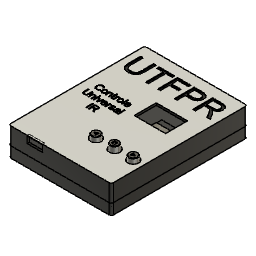
NOVACASEEMBARCADOS v11 (Autodesk Fusion 360 design; units mm, degrees)
Autodesk Fusion 360 part; units mm, degrees
sketch "Esboço1" plane through (0, 0, 0) normal (0, 0, 1) x (1, 0, 0)
  line L0 (-44.75, 0) -> (-44.75, 60)
  line L1 (-44.75, 0) -> (-44.75, -60)
  line L2 (-44.75, -60) -> (44.75, -60)
  line L3 (44.75, -60) -> (44.75, 60)
  line L4 (44.75, 60) -> (-44.75, 60)
  dimension "d2" = 44.75
  dimension "d3" = 60
  dimension "d4" = 60
  dimension "d5" = 89.5
  constraint perpendicular L1 L2
  constraint perpendicular L2 L3
  constraint perpendicular L0 L4
  measures "d2" distance of origin L0.start
  measures "d3" distance of L0.start L0.end
  measures "d4" distance of L0.start L1.end
  measures "d5" distance of L1.end L2.end
extrude "Extrusão1" add sketch "Esboço1" along normal blind 1.5 makes body 1
sketch "Esboço2" plane through (0, 0, 1.5) normal (0, 0, 1) x (-1, 0, 0)
  line L0 (44.75, -60) -> (44.75, 60)
  line L1 (44.75, 60) -> (-44.75, 60)
  line L2 (-44.75, 60) -> (-44.75, -60)
  line L3 (-44.75, -60) -> (44.75, -60)
  line L4 (-40.75, 36) -> (-34.75, 36)
  line L5 (-40.75, 36) -> (-40.75, 30)
  line L6 (-34.75, 36) -> (-34.75, 30)
  line L7 (-34.75, 30) -> (-40.75, 30)
  line L8 (-23.75, 36) -> (-17.75, 36)
  line L9 (-23.75, 36) -> (-23.75, 30)
  line L10 (-17.75, 36) -> (-17.75, 30)
  line L11 (-17.75, 30) -> (-23.75, 30)
  line L12 (-0.75, 30) -> (-6.75, 30)
  line L13 (-6.75, 36) -> (-6.75, 30)
  line L14 (-6.75, 36) -> (-0.75, 36)
  line L15 (-0.75, 36) -> (-0.75, 30)
  line L16 (-31.75, 0) -> (-3.75, 0)
  line L17 (-3.75, 0) -> (-3.75, -27)
  line L18 (-31.75, 0) -> (-31.75, -27)
  line L19 (-31.75, -27) -> (-3.75, -27)
  line L20 (36.75, 57) -> (8.75, 57)
  line L21 (8.75, 57) -> (8.75, 6)
  line L22 (36.75, 57) -> (36.75, 6)
  line L23 (36.75, 6) -> (8.75, 6)
  dimension "d10" = 6
  dimension "d11" = 6
  dimension "d12" = 11
  dimension "d13" = 6
  dimension "d15" = 6
  dimension "d18" = 28
  dimension "d19" = 27
  dimension "d22" = 28
  dimension "d23" = 51
  constraint perpendicular L4 L5
  constraint perpendicular L4 L6
  constraint perpendicular L5 L7
  constraint perpendicular L8 L10
  constraint perpendicular L9 L11
  constraint perpendicular L14 L15
  constraint perpendicular L12 L13
  constraint perpendicular L17 L19
  constraint perpendicular L20 L21
  constraint perpendicular L20 L22
  constraint perpendicular L21 L23
  measures "d10" distance of L4.start L4.end
  measures "d11" distance of L4.start L5.end
  measures "d12" distance of L4.end L8.start
  measures "d13" distance of L8.start L8.end
  measures "d15" distance of L13.start L14.end
  measures "d18" distance of L16.start L16.end
  measures "d19" distance of L16.end L17.end
  measures "d22" distance of L20.start L20.end
  measures "d23" distance of L20.end L21.end
extrude "Extrusão2" add sketch "Esboço2" along normal blind 16.5 contours L20 L21 L22 L23 bodies 1
extrude "Extrusão3" add sketch "Esboço2" along normal blind 3.5 contours L16 L17 L18 L19 bodies 1
extrude "Extrusão4" add sketch "Esboço2" along normal blind 3.5 contours L4 L5 L6 L7 | L8 L9 L10 L11 | L12 L13 L14 L15 bodies 1
sketch "Esboço3" plane through (0, 0, 5) normal (0, 0, 1) x (-1, 0, 0)
  line L0 (-31.75, 0) -> (-31.75, -27)
  line L1 (-31.75, -27) -> (-3.75, -27)
  line L2 (-3.75, -27) -> (-3.75, 0)
  line L3 (-3.75, 0) -> (-31.75, 0)
  line L4 (-29.75, -4.5) -> (-5.25, -4.5)
  line L5 (-5.25, -4.5) -> (-5.25, -20.5)
  line L6 (-5.25, -20.5) -> (-29.75, -20.5)
  line L7 (-29.75, -20.5) -> (-29.75, -4.5)
  dimension "d32" = 24.5
  dimension "d33" = 16
  constraint perpendicular L4 L5
  constraint perpendicular L4 L7
  measures "d32" distance of L4.start L4.end
  measures "d33" distance of L4.end L5.end
extrude "Extrusão5" add sketch "Esboço3" along normal blind 2 contours L4 L5 L6 L7 bodies 1
sketch "Esboço4" plane through (0, 0, 1.5) normal (0, 0, 1) x (-1, 0, 0)
sketch "Esboço5" plane through (0, 0, 5) normal (0, 0, 1) x (-1, 0, 0)
  line L0 (-40.75, 36) -> (-40.75, 30)
  line L1 (-40.75, 30) -> (-34.75, 30)
  line L2 (-34.75, 30) -> (-34.75, 36)
  line L3 (-34.75, 36) -> (-40.75, 36)
  circle A0 centre (-3.75, 33) radius 1.5
  circle A1 centre (-20.75, 33) radius 1.5
  circle A2 centre (-37.75, 33) radius 1.5
  dimension "d40" = 3
  dimension "d41" = 3
  dimension "d42" = 3
  measures "d40" diameter of A0
  measures "d41" diameter of A1
  measures "d42" diameter of A2
extrude "Extrusão6" add sketch "Esboço5" along normal blind 2 contours A0 | A2 bodies 1
extrude "Extrusão7" add sketch "Esboço5" along normal blind 3 contours A1 bodies 1
chamfer "Chanfro1" distance 0.25 distance2 3 1 edges at (22.1485, -32.4576, 8) measured on face at (20.7773, -33.3643, 8) on bodies 1
sketch "Esboço7" plane through (0, -57, 0) normal (0, -1, 0) x (1, 0, 0)
  line L0 (-36.75, 1.5) -> (-8.75, 1.5)
  line L1 (-8.75, 1.5) -> (-8.75, 18)
  line L2 (-8.75, 18) -> (-36.75, 18)
  line L3 (-36.75, 18) -> (-36.75, 1.5)
  line L4 (-26.75, 18) -> (-19.75, 18)
  line L5 (-27.75, 17) -> (-26.75, 18)
  line L6 (-27.75, 17) -> (-26.25, 16)
  line L7 (-26.25, 16) -> (-21.25, 16)
  line L8 (-19.75, 18) -> (-18.75, 17)
  line L9 (-18.75, 17) -> (-20, 16)
  line L10 (-20, 16) -> (-21.25, 16)
  line L11 (-27.75, 17) -> (-26.25, 16)
  dimension "d49" = 10
  dimension "d50" = 7
  dimension "d55" = 5
  constraint parallel L2 L4
  constraint horizontal L7
  measures "d49" distance of L2.end L4.start
  measures "d50" distance of L4.start L4.end
  measures "d55" distance of L6.end L7.end
extrude "Extrusão8" cut sketch "Esboço7" against normal blind 5 contours L2 L4 L5 L6 L7 L8 L9 L10 L11 bodies 1
sketch "Esboço8" plane through (0, 0, 1.5) normal (0, 0, 1) x (-1, 0, 0)
sketch "Esboço9" plane through (0, 0, 0) normal (0, 0, 1) x (1, 0, 0)
  line L0 (164.75, -60) -> (75.25, -60)
  line L1 (75.25, -60) -> (75.25, 60)
  line L2 (164.75, 60) -> (164.75, -60)
  line L3 (75.25, 60) -> (164.75, 60)
  line L4 (73.25, -62) -> (73.25, 62)
  line L5 (73.25, 62) -> (166.75, 62)
  line L6 (166.75, 62) -> (166.75, -62)
  line L7 (166.75, -62) -> (73.25, -62)
  dimension "d61" = -2
  constraint horizontal L3
  constraint vertical L2
  constraint horizontal L0
  constraint vertical L1
extrude "Extrusão9" add sketch "Esboço9" along normal blind 2 separate body contours L0 L1 L2 L3 makes body 2
extrude "Extrusão11" add sketch "Esboço9" along normal blind 9.75 bodies 2
sketch "Esboço10" plane through (0, 0, 9.75) normal (0, 0, 1) x (-1, 0, 0)
  line L0 (-75.25, 60) -> (-75.25, -60)
  line L1 (-75.25, -60) -> (-164.75, -60)
  line L2 (-164.75, -60) -> (-164.75, 60)
  line L3 (-164.75, 60) -> (-75.25, 60)
  line L4 (-166.75, 62) -> (-166.75, -62)
  line L5 (-166.75, -62) -> (-73.25, -62)
  line L6 (-73.25, -62) -> (-73.25, 62)
  line L7 (-73.25, 62) -> (-166.75, 62)
  line L8 (-74.25, 61) -> (-74.25, -61)
  line L9 (-74.25, -61) -> (-165.75, -61)
  line L10 (-165.75, -61) -> (-165.75, 61)
  line L11 (-165.75, 61) -> (-74.25, 61)
extrude "Extrusão12" cut sketch "Esboço10" against normal blind 3 contours L8 L9 L10 L11 bodies 2
sketch "Esboço11" plane through (0, 0, 0) normal (0, 0, 1) x (1, 0, 0)
  line L0 (203.25, 62) -> (296.75, 62)
  line L1 (296.75, 62) -> (296.75, -62)
  line L2 (296.75, -62) -> (203.25, -62)
  line L3 (203.25, -62) -> (203.25, 62)
  line L4 (294.75, -60) -> (205.25, -60)
  line L5 (205.25, -60) -> (205.25, 60)
  line L6 (205.25, 60) -> (294.75, 60)
  line L7 (294.75, 60) -> (294.75, -60)
  dimension "d71" = 2
  constraint horizontal L0
  constraint vertical L1
  constraint horizontal L2
  constraint vertical L3
extrude "Extrusão13" add sketch "Esboço11" along normal blind 2 separate body contours L4 L5 L6 L7 makes body 3
extrude "Extrusão14" add sketch "Esboço11" along normal blind 12.75 bodies 3
sketch "Esboço12" plane through (0, 0, 12.75) normal (0, 0, 1) x (-1, 0, 0)
  line L0 (-205.25, -60) -> (-294.75, -60)
  line L1 (-294.75, -60) -> (-294.75, 60)
  line L2 (-294.75, 60) -> (-205.25, 60)
  line L3 (-205.25, 60) -> (-205.25, -60)
  line L4 (-203.25, 62) -> (-296.75, 62)
  line L5 (-296.75, 62) -> (-296.75, -62)
  line L6 (-296.75, -62) -> (-203.25, -62)
  line L7 (-203.25, -62) -> (-203.25, 62)
  line L8 (-203.25, -62) -> (-296.75, -62)
  line L9 (-296.75, -62) -> (-296.75, 62)
  line L10 (-296.75, 62) -> (-203.25, 62)
  line L11 (-203.25, 62) -> (-203.25, -62)
  line L12 (-295.75, -61) -> (-295.75, 61)
  line L13 (-295.75, 61) -> (-204.25, 61)
  line L14 (-204.25, 61) -> (-204.25, -61)
  line L15 (-204.25, -61) -> (-295.75, -61)
  dimension "d76" = 1
  constraint horizontal L8
  constraint vertical L9
  constraint horizontal L10
  constraint vertical L11
  constraint coincident L4.end L5.start
  constraint coincident L6.end L7.start
extrude "Extrusão15" cut sketch "Esboço12" against normal blind 3 contours L4 L5 L6 L7 L8 L9 L10 L11 bodies 3
move_body "Alinhar1" bodies 1 to x (1, 0, 0) y (0, 1, 0) z (0, 0, 1) at (120, 0, 0)
move_body "Mover1" bodies 3 to x (-1, 0, 0) y (0, 1, 0) z (0, 0, -1) at (591.5, 0, 25.5)
move_body "Alinhar2" bodies 3 to x (1, 0, 0) y (0, 1, 0) z (0, 0, 1) at (-221.5, 0, -6)
sketch "Esboço13" plane through (0, 0, 19.5) normal (0, 0, 1) x (-1, 0, 0)
  line L0 (-73.25, 62) -> (-166.75, 62)
  line L1 (-166.75, 62) -> (-166.75, -62)
  line L2 (-166.75, -62) -> (-73.25, -62)
  line L3 (-73.25, -62) -> (-73.25, 62)
  line L4 (-151.75, -2.5) -> (-123.25, -2.5)
  line L5 (-123.25, -2.5) -> (-123.25, -22.5)
  line L6 (-123.25, -22.5) -> (-151.75, -22.5)
  line L7 (-151.75, -22.5) -> (-151.75, -2.5)
  circle A0 centre (-123.75, 33) radius 5
  circle A1 centre (-140.75, 33) radius 5
  circle A2 centre (-157.75, 33) radius 5
  dimension "d81" = 10
  dimension "d82" = 10
  dimension "d83" = 10
  measures "d81" diameter of A0
  measures "d82" diameter of A1
  measures "d83" diameter of A2
extrude "Extrusão16" add sketch "Esboço13" against normal blind 2 separate body contours L4 L5 L6 L7 | A0 | A1 | A2 makes body 4 at (140.1411, -30.9517, 19.5) makes body 5 at (157.1411, -30.9517, 19.5) makes body 6 at (132.75, 15.8333, 19.5) makes body 7 at (122.4284, -33.696, 19.5)
extrude "Extrusão17" add 4 faces at (140.1411, -30.9517, 19.5) (122.4284, -33.696, 19.5) (157.1411, -30.9517, 19.5) (132.75, 15.8333, 19.5) along direction (0, 0, -1) blind 2 on bodies 4 5 6 7 bodies 3 4 5 6 7
extrude "Extrusão18" cut sketch "Esboço13" against normal blind 3 contours L4 L5 L6 L7 | A0 | A1 | A2 bodies 3
fillet "Arredondamento1" radius 2 2 edges at (166.75, -62, 4.875) (166.75, -62, 14.625) on bodies 2 3
fillet "Arredondamento2" radius 2 2 edges at (73.25, -62, 4.875) (73.25, -62, 14.625) on bodies 2 3
fillet "Arredondamento3" radius 2 2 edges at (166.75, 62, 4.875) (166.75, 62, 14.625) on bodies 2 3
fillet "Arredondamento4" radius 2 2 edges at (73.25, 62, 4.875) (73.25, 62, 14.625) on bodies 2 3
sketch "Esboço14" plane through (0, 0, 19.5) normal (0, 0, 1) x (-1, 0, 0)
  arc A0 (-75.25, -62) -> (-73.25, -60) centre (-75.25, -60) ccw
  line L0 (-73.25, -60) -> (-73.25, 60)
  arc A1 (-73.25, 60) -> (-75.25, 62) centre (-75.25, 60) ccw
  line L1 (-75.25, 62) -> (-164.75, 62)
  arc A2 (-164.75, 62) -> (-166.75, 60) centre (-164.75, 60) ccw
  line L2 (-166.75, 60) -> (-166.75, -60)
  arc A3 (-166.75, -60) -> (-164.75, -62) centre (-164.75, -60) ccw
  line L3 (-164.75, -62) -> (-75.25, -62)
  circle A4 centre (-140.75, 33) radius 5
  line L4 (-123.25, -2.5) -> (-123.25, -22.5)
  line L5 (-123.25, -22.5) -> (-151.75, -22.5)
  line L6 (-151.75, -22.5) -> (-151.75, -2.5)
  line L7 (-151.75, -2.5) -> (-123.25, -2.5)
  circle A5 centre (-123.75, 33) radius 5
  circle A6 centre (-157.75, 33) radius 5
  line L8 (-78.6403, -28.775) -> (-161.6972, -28.775) construction
  line L9 (-161.6972, -28.775) -> (-161.6972, -57.452) construction
  line L10 (-161.6972, -57.452) -> (-78.6403, -57.452) construction
  line L11 (-78.6403, -57.452) -> (-78.6403, -28.775) construction
  line L12 (-79.2776, 23.0559) -> (-116.8762, 23.0559) construction
  line L13 (-116.8762, 23.0559) -> (-116.8762, -21.9776) construction
  line L14 (-116.8762, -21.9776) -> (-79.2776, -21.9776) construction
  line L15 (-79.2776, -21.9776) -> (-79.2776, 23.0559) construction
  dimension "d98" = 18
  dimension "d99" = 6
  text T0 "UTFPR" font "Arial" height 18 align centre middle in box 83.0569 x 28.6769 at (-78.6403, -28.775) x (-1, 0) y (0, -1) spacing 1 kerned
  text T1 "Controle\nUniversal\nIR" font "Arial" height 6 align centre middle in box 37.5986 x 45.0334 at (-79.2776, 23.0559) x (-1, 0) y (0, -1) spacing 1 kerned
extrude "Extrusão19" cut sketch "Esboço14" against normal blind 1 text T1 T0 bodies 3
sketch "Esboço15" plane through (0, 62, 0) normal (0, 1, 0) x (-1, 0, 0)
  line L0 (-75.25, 9.75) -> (-75.25, 19.5)
  line L1 (-75.25, 19.5) -> (-164.75, 19.5)
  line L2 (-164.75, 19.5) -> (-164.75, 9.75)
  line L3 (-164.75, 9.75) -> (-75.25, 9.75)
  line L4 (-79.25, 6) -> (-104.25, 6)
  line L5 (-79.25, 6) -> (-79.25, 16)
  line L6 (-104.25, 6) -> (-104.25, 16)
  line L7 (-104.25, 16) -> (-79.25, 16)
  dimension "d104" = 25
  dimension "d105" = 10
  constraint perpendicular L3 L5
  constraint perpendicular L4 L6
  constraint perpendicular L5 L7
  measures "d104" distance of L4.start L4.end
  measures "d105" distance of L4.start L5.end
extrude "Extrusão20" cut sketch "Esboço15" against normal blind 2 contours L3 L4 L5 L6 | L3 L5 L6 L7 bodies 2 3
sketch "Esboço16" plane through (0, -62, 0) normal (0, -1, 0) x (1, 0, 0)
  line L0 (75.25, 19.5) -> (75.25, 9.75)
  line L1 (75.25, 9.75) -> (164.75, 9.75)
  line L2 (164.75, 9.75) -> (164.75, 19.5)
  line L3 (164.75, 19.5) -> (75.25, 19.5)
  line L4 (90, 18) -> (90, 14)
  line L5 (90, 14) -> (104, 14)
  line L6 (104, 14) -> (104, 19)
  line L7 (104, 19) -> (90, 19)
  line L8 (90, 19) -> (90, 18)
  constraint vertical L4
  constraint perpendicular L4 L5
  constraint perpendicular L5 L6
  constraint perpendicular L6 L7
  constraint perpendicular L7 L8
extrude "Extrusão21" cut sketch "Esboço16" against normal blind 2 contours L4 L5 L6 L7 L8 bodies 3
move_body "Alinhar3" bodies 3 to x (1, 0, 0) y (0, 1, 0) z (0, 0, 1) at (0, 0, -19.5)
move_body "Mover2" bodies 3 to x (-1, 0, 0) y (0, 1, 0) z (0, 0, -1) at (286.5, 0, -25.5)
move_body "Mover3" bodies 3 to x (1, 0, 0) y (0, 1, 0) z (0, 0, 1) at (90, 0, 0)
extrude "Extrusão22" add 1 faces at (302.5833, -20, -15.75) along direction (0, 0, 1) blind 4 on bodies 3 bodies 3
extrude "Extrusão23" add 1 faces at (211.0833, 20, -12.75) along direction (0, 0, 1) blind 4 on bodies 3 bodies 3
sketch "Esboço17" plane through (0, -62, 0) normal (0, -1, 0) x (1, 0, 0)
  line L0 (272.5, -20) -> (286.5, -20)
  line L1 (286.5, -20) -> (286.5, -25)
  line L2 (286.5, -25) -> (272.5, -25)
  line L3 (272.5, -25) -> (272.5, -20)
  line L4 (301.25, -25.5) -> (301.25, -11.75)
  line L5 (301.25, -11.75) -> (211.75, -11.75)
  line L6 (211.75, -11.75) -> (211.75, -25.5)
  line L7 (211.75, -25.5) -> (301.25, -25.5)
extrude "Extrusão24" add 1 faces at (105.0833, 20, 0) along direction (0, 0, -1) blind 5 on bodies 1 bodies 1
move_body "Mover4" bodies 1 to x (1, 0, 0) y (0, 1, 0) z (0, 0, 1) at (0, 0, 5)
extrude "Extrusão25" add 1 faces at (302.5833, -20, -11.75) along direction (0, 0, 1) blind 4 on bodies 3 bodies 3
extrude "Extrusão26" add 1 faces at (211.0833, 20, -8.75) along direction (0, 0, 1) blind 4 on bodies 3 bodies 3
move_body "Alinhar5" bodies 3 to x (1, 0, 0) y (0, 1, 0) z (0, 0, 1) at (-45, 0, 17.5)
move_body "Mover7" bodies 3 to x (-1, 0, 0) y (0, 1, 0) z (0, 0, -1) at (329.5, 0, -16)
move_body "Mover8" bodies 3 to x (1, 0, 0) y (0, 1, 0) z (0, 0, 1) at (2, 0, 35.5)
extrude "Extrusão27" cut 1 faces at (73.9167, -20, 9.75) along direction (0, 0, 1) blind 2 on bodies 3 bodies 3
extrude "Extrusão28" cut 1 faces at (165.4167, 20, 6.75) along direction (0, 0, 1) blind 2 on bodies 3 bodies 3
move_body "Mover9" bodies 3 to x (1, 0, 0) y (0, 1, 0) z (0, 0, 1) at (0, 0, -2)
extrude "Extrusão29" cut 1 faces at (94.6667, -61.3333, 20) along direction (0, 0, -1) blind 2 on bodies 3 bodies 3
extrude "Extrusão30" add 1 faces at (94.6667, -61.3333, 18) along direction (0, 0, 1) blind 1 on bodies 3 bodies 3
sketch "Esboço18" plane through (0, 0, 0) normal (0, 0, 1) x (1, 0, 0)
  circle A0 centre (20, -20) radius 4.5
  circle A1 centre (-10, -20) radius 4.5
  circle A2 centre (-35, -20) radius 4.5
  dimension "d128" = 9
  dimension "d129" = 9
  dimension "d130" = 9
  measures "d128" diameter of A0
  measures "d129" diameter of A1
  measures "d130" diameter of A2
sketch "Esboço19" plane through (0, 0, 20) normal (0, 0, 1) x (-1, 0, 0)
  line L0 (9, 19) -> (11, 19)
  line L1 (11, 19) -> (11, 21)
  line L2 (11, 21) -> (9, 21)
  line L3 (9, 21) -> (9, 19)
  line L4 (9, 19) -> (11, 21) construction
  line L5 (11, 19) -> (9, 21) construction
  line L6 (-19, 19) -> (-19, 21)
  line L7 (34, 21) -> (34, 19)
  line L8 (34, 19) -> (36, 20)
  line L9 (36, 20) -> (34, 21)
  line L10 (-19, 19) -> (-21, 20)
  line L11 (-21, 20) -> (-19, 21)
  circle A0 centre (-20, 20) radius 4.5
  circle A1 centre (35, 20) radius 4.5
  circle A2 centre (10, 20) radius 4.5
  point P0 (10, 20)
  point P1 (-20, 20)
  point P2 (35, 20)
  constraint horizontal L0
  constraint perpendicular L0 L1
  constraint parallel L0 L2
  constraint parallel L1 L3
  constraint coincident L4 P0
  constraint coincident L5 P0
sketch "Esboço20" plane through (0, 0, 0) normal (0, 0, -1) x (1, 0, 0)
  circle A0 centre (-10, 20) radius 4.5
  circle A1 centre (-10, 20) radius 2.25
  circle A2 centre (20, 20) radius 2.25
  circle A3 centre (-35, 20) radius 2.25
  dimension "d141" = 4.5
  dimension "d142" = 4.5
  dimension "d143" = 4.5
  constraint concentric A0 A1
  measures "d141" diameter of A1
  measures "d142" diameter of A2
  measures "d143" diameter of A3
sketch "Esboço21" plane through (0, 0, 0) normal (0, 0, 1) x (1, 0, 0)
  circle A0 centre (25, 25) radius 4
  circle A1 centre (10, 25) radius 4
  circle A2 centre (-10, 25) radius 4
  dimension "d148" = 8
  dimension "d149" = 8
  dimension "d150" = 8
  measures "d148" diameter of A0
  measures "d149" diameter of A1
  measures "d150" diameter of A2
extrude "Extrusão36" add sketch "Esboço21" along normal blind 20 separate body contours A1 makes body 8
extrude "Extrusão37" add sketch "Esboço21" along normal blind 20 separate body contours A0 | A2 makes body 9 at (-6.005, 24.8006, 13.3333) makes body 10 at (28.995, 24.8006, 13.3333)
fillet "Arredondamento7" radius 0.5 1 edges at (-13.7293, 23.5535, 20) on bodies 9
fillet "Arredondamento8" radius 0.5 1 faces at (9.7033, 26.2999, 20) on bodies 8
fillet "Arredondamento9" radius 0.5 1 edges at (21.2707, 23.5535, 20) on bodies 10
sketch "Esboço22" plane through (0, 0, 20) normal (0, 0, 1) x (-1, 0, 0)
  circle A0 centre (-10, -25) radius 3.5
  line L0 (-8.5, -23.4828) -> (-11.5, -23.4828)
  line L1 (-11.5, -23.4828) -> (-11.5, -26.5172)
  line L2 (-11.5, -26.5172) -> (-8.5, -26.5172)
  line L3 (-8.5, -26.5172) -> (-8.5, -23.4828)
  line L4 (-8.5, -23.4828) -> (-11.5, -26.5172) construction
  line L5 (-11.5, -23.4828) -> (-8.5, -26.5172) construction
  line L6 (-23.75, -23.4597) -> (-23.75, -26.5403)
  line L7 (-23.75, -26.5403) -> (-26.75, -25)
  line L8 (-26.75, -25) -> (-23.75, -23.4597)
  line L9 (8.75, -23.5) -> (8.75, -26.5)
  line L10 (8.75, -26.5) -> (11.75, -25)
  line L11 (11.75, -25) -> (8.75, -23.5)
  point P0 (-10, -25)
  point P1 (-25.25, -25)
  point P2 (10.25, -25)
  dimension "d161" = 3
  constraint horizontal L0
  constraint perpendicular L0 L1
  constraint parallel L0 L2
  constraint parallel L1 L3
  constraint coincident L4 P0
  constraint coincident L5 P0
  constraint coincident P0 A0.centre
  measures "d161" distance of L1.end L2.end
extrude "Extrusão38" cut sketch "Esboço22" against normal blind 1 contours L0 L1 L2 L3 | L6 L7 L8 | L9 L10 L11 bodies 8 9 10
sketch "Esboço23" plane through (0, 0, 0) normal (0, 0, 1) x (1, 0, 0)
  circle A0 centre (10, 25) radius 2.25
  circle A1 centre (25, 25) radius 2.25
  dimension "d165" = 4.5
  dimension "d166" = 4.5
  measures "d165" diameter of A0
  measures "d166" diameter of A1
sketch "Esboço24" plane through (0, 0, 0) normal (0, 0, 1) x (1, 0, 0)
  line L0 (-25, -45) -> (-16.5, -45)
  line L1 (-16.5, -45) -> (-16.5, -36.5)
  line L2 (-25, -45) -> (-25, -36.5)
  line L3 (-25, -36.5) -> (-16.5, -36.5)
  line L4 (-17.25, -37.2158) -> (-24.25, -37.2158)
  line L5 (-24.25, -37.2158) -> (-24.25, -44.2842)
  line L6 (-24.25, -44.2842) -> (-17.25, -44.2842)
  line L7 (-17.25, -44.2842) -> (-17.25, -37.2158)
  line L8 (-17.25, -37.2158) -> (-24.25, -44.2842) construction
  line L9 (-24.25, -37.2158) -> (-17.25, -44.2842) construction
  point P0 (-20.75, -40.75)
  dimension "d174" = 8.5
  dimension "d175" = 8.5
  dimension "d176" = 7
  constraint horizontal L0
  constraint perpendicular L0 L1
  constraint perpendicular L0 L2
  constraint perpendicular L1 L3
  constraint horizontal L4
  constraint perpendicular L4 L5
  constraint parallel L4 L6
  constraint parallel L5 L7
  constraint coincident L8 P0
  constraint coincident L9 P0
  measures "d174" distance of L0.start L0.end
  measures "d175" distance of L0.end L1.end
  measures "d176" distance of L5.end L6.end
extrude "Extrusão42" add sketch "Esboço24" along normal blind 3 separate body makes body 11
sketch "Esboço25" plane through (0, 0, 3) normal (0, 0, 1) x (-1, 0, 0)
  line L0 (17.25, 37.2158) -> (17.25, 44.2842)
  line L1 (17.25, 44.2842) -> (24.25, 44.2842)
  line L2 (24.25, 44.2842) -> (24.25, 37.2158)
  line L3 (24.25, 37.2158) -> (17.25, 37.2158)
  line L4 (25, 45) -> (16.5, 45)
  line L5 (16.5, 45) -> (16.5, 36.5)
  line L6 (16.5, 36.5) -> (25, 36.5)
  line L7 (25, 36.5) -> (25, 45)
  line L8 (25, 36.5) -> (16.5, 36.5)
  line L9 (16.5, 45) -> (16.5, 36.5)
  line L10 (16.5, 45) -> (25, 45)
  line L11 (25, 45) -> (25, 36.5)
  constraint coincident L6.end L7.start
  constraint coincident L5.end L6.start
  constraint coincident L4.end L5.start
  constraint coincident L4.start L7.end
extrude "Extrusão44" cut 1 faces at (-24.75, -39.5719, 3) along direction (0, 0, -1) blind 0.5 on bodies 11 bodies 11
sketch "Esboço26" plane through (0, 0, 2.5) normal (0, 0, 1) x (-1, 0, 0)
  line L0 (17.25, 37.2158) -> (17.25, 44.2842)
  line L1 (17.25, 44.2842) -> (24.25, 44.2842)
  line L2 (24.25, 44.2842) -> (24.25, 37.2158)
  line L3 (24.25, 37.2158) -> (17.25, 37.2158)
  line L4 (25, 45) -> (16.5, 45)
  line L5 (16.5, 45) -> (16.5, 36.5)
  line L6 (16.5, 36.5) -> (25, 36.5)
  line L7 (25, 36.5) -> (25, 45)
  line L8 (25, 36.5) -> (16.5, 36.5)
  line L9 (16.5, 36.5) -> (16.5, 45)
  line L10 (25, 45) -> (16.5, 45)
  line L11 (25, 45) -> (25, 36.5)
  constraint coincident L6.end L7.start
  constraint coincident L5.end L6.start
  constraint coincident L4.end L5.start
  constraint coincident L4.start L7.end
extrude "Extrusão45" add sketch "Esboço26" along normal blind 0.5 separate body contours L0 L1 L2 L3 makes body 12
extrude "Extrusão46" add 1 faces at (-24.75, -39.5719, 2.5) along direction (0, 0, 1) blind 0.5 on bodies 11 bodies 11 12
extrude "Extrusão48" cut 3 faces at (-10.2967, 26.2999, 0) (9.7033, 26.2999, 0) (26.146, 24.0546, 0) along direction (0, 0, 1) blind 3 on bodies 8 9 10 bodies 8 9 10
move_body "Alinhar7" bodies 9 to x (1, 0, 0) y (0, 1, 0) z (0, 0, 1) at (-10.75, -65.75, 0)
copy_body "Copiar e colar corpos1" bodies 11 makes body 13
move_body "Mover10" bodies 13 to x (1, 0, 0) y (0, 1, 0) z (0, 0, 1) at (16, 0, 0)
copy_body "Copiar e colar corpos2" bodies 11 makes body 14
move_body "Mover11" bodies 14 to x (1, 0, 0) y (0, 1, 0) z (0, 0, 1) at (36, 0, 0)
move_body "Alinhar8" bodies 8 to x (1, 0, 0) y (0, 1, 0) z (0, 0, 1) at (-14.75, -65.75, 0)
move_body "Alinhar9" bodies 10 to x (1, 0, 0) y (0, 1, 0) z (0, 0, 1) at (-9.75, -65.75, 0)
combine "Combinar1" operation add target body 10 tool bodies 14
combine "Combinar2" operation add target body 13 tool bodies 8
combine "Combinar3" operation add target body 11 tool bodies 9
extrude "Extrusão49" add 1 faces at (-8.75, -39.5719, 0) along direction (0, 0, -1) blind 0.9 on bodies 13 bodies 13
extrude "Extrusão50" add 1 faces at (-8.75, -39.5719, -0.9) along direction (0, 0, -1) blind 2 on bodies 13 bodies 13
extrude "Extrusão51" add 2 faces at (11.25, -39.5719, 0) (-24.75, -39.5719, 0) along direction (0, 0, -1) blind 2 on bodies 10 11 bodies 10 11
extrude "Extrusão52" add 3 faces at (-23.9754, -37.384, 3) (-7.9754, -37.384, 3) (18.4754, -37.384, 3) along direction (0, 0, 1) blind 9 on bodies 10 11 13 bodies 11 10 13
move_body "Alinhar10" bodies 10 to x (1, 0, 0) y (0, 1, 0) z (0, 0, 1) at (142.5, 7.75, 9.5)
move_body "Alinhar11" bodies 13 to x (1, 0, 0) y (0, 1, 0) z (0, 0, 1) at (145.5, 7.75, 10.5)
move_body "Alinhar12" bodies 11 to x (1, 0, 0) y (0, 1, 0) z (0, 0, 1) at (144.5, 7.75, 9.5)
equation "d3 = ( 120 / 2 ) * 1 mm"
equation "d24 = 18 mm - 1.5 mm"
equation "d26 = 5 mm - 1.5 mm"
equation "d28 = 5 mm - 1.5 mm"
equation "d34 = 7 mm - 5 mm"
equation "d43 = 7 mm - 5 mm"
equation "d45 = 8 mm - 5 mm"
